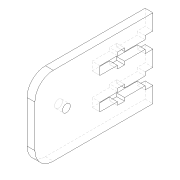
# Autodesk Inventor part: axel mount (3mm shaft)
Saved by Autodesk Inventor 2016 (Build 200138000, 138)
## iProperties
Created: 2014-07-12
Part Number: axel mount (3mm shaft)
Material: Plywood, Finish
Document SubType Name: Modeling
Designer: Sebastian
Density: 0.552 g/cm^3
Appearance: Plywood - New
Description: http://www.wickes.co.uk/Wickes-Non-Structural-Hardwood-Plywood-3-6x607x1829mm/p/110513
Author: Sebastian
Autodesk Inventor part; units mm, degrees
ref_plane "YZ Plane" through (0, 0, 0) normal (1, 0, 0) x (0, 1, 0)
ref_plane "XZ Plane" through (0, 0, 0) normal (0, 1, 0) x (-1, 0, 0)
ref_plane "XY Plane" through (0, 0, 0) normal (0, 0, 1) x (1, 0, 0)
sketch "Sketch1" plane through (0, 0, 0) normal (1, 0, 0) x (0, 1, 0)
  line L0 (0, 0) -> (45, 0)
  line L1 (45, 0) -> (45, -30)
  line L2 (45, -30) -> (0, -30)
  line L3 (0, -30) -> (0, 0)
  dimension "d0" = 45
  dimension "d1" = 30
  constraints: 8 end point, 2 parallel, 1 horizontal, 1 perpendicular
  measures "d0" distance of L1.end L2.end
  measures "d1" distance of L0.end L1.end
extrude "Extrusion1" add sketch "Sketch1" along normal blind 3
sketch "Sketch2" plane through (3, 0, 0) normal (1, 0, 0) x (0, 0, -1)
  line L0 (30, 45) -> (0, 45) projected
  line L1 (6, 45) -> (12, 45)
  line L2 (12, 45) -> (12, 42)
  line L3 (6, 42) -> (6, 45)
  line L4 (0, 45) -> (0, 0) projected
  line L5 (18, 45) -> (24, 45)
  line L6 (24, 45) -> (24, 42)
  line L7 (18, 42) -> (18, 45)
  line L8 (30, 0) -> (30, 45) projected
  line L9 (6, 42) -> (7.4, 42)
  line L10 (7.4, 42) -> (7.4, 34.2)
  line L11 (7.4, 34.2) -> (6.2, 34.2)
  line L12 (6.2, 34.2) -> (6.2, 31.45)
  line L13 (6.2, 31.45) -> (7.4, 31.45)
  line L14 (7.4, 31.45) -> (7.4, 24.8)
  line L15 (7.4, 24.8) -> (10.6, 24.8)
  line L16 (10.6, 24.8) -> (10.6, 31.45)
  line L17 (10.6, 31.45) -> (11.8, 31.45)
  line L18 (11.8, 31.45) -> (11.8, 34.2)
  line L19 (11.8, 34.2) -> (10.6, 34.2)
  line L20 (10.6, 42) -> (12, 42)
  line L21 (10.6, 34.2) -> (10.6, 42)
  line L22 (18, 42) -> (19.4, 42)
  line L23 (19.4, 42) -> (19.4, 34.2)
  line L24 (19.4, 34.2) -> (18.2, 34.2)
  line L25 (18.2, 34.2) -> (18.2, 31.45)
  line L26 (18.2, 31.45) -> (19.4, 31.45)
  line L27 (19.4, 24.8) -> (19.4, 31.45)
  line L28 (19.4, 24.8) -> (22.6, 24.8)
  line L29 (22.6, 24.8) -> (22.6, 31.45)
  line L30 (22.6, 31.45) -> (23.8, 31.45)
  line L31 (23.8, 31.45) -> (23.8, 34.2)
  line L32 (23.8, 34.2) -> (22.6, 34.2)
  line L33 (22.6, 42) -> (24, 42)
  line L34 (22.6, 42) -> (22.6, 34.2)
  dimension "d4" = 6
  dimension "d6" = 6
  dimension "d18" = 6
  dimension "d19" = 3
  dimension "d20" = 6
  dimension "d21" = 6
  dimension "d22" = 1.4
  dimension "d23" = 7.8
  dimension "d24" = 1.2
  dimension "d25" = 2.75
  dimension "d26" = 1.2
  dimension "d27" = 6.65
  dimension "d28" = 3.2
  dimension "d29" = 1.2
  dimension "d30" = 1.4
  dimension "d31" = 1.2
  dimension "d32" = 3.2
  dimension "d33" = 1.2
  dimension "d34" = 20.2
  constraints: 64 end point, 27 point on line, 15 perpendicular, 4 parallel, 3 horizontal
  measures "d4" distance of L2.end L3.start
  measures "d6" distance between parallel lines of L3 L4
  measures "d18" distance of L6.end L7.start
  measures "d19" distance of L5.end L6.end
  measures "d20" distance between parallel lines of L8 L6
  measures "d21" distance between parallel lines of L7 L2
  measures "d22" distance of L3.start L9.end
  measures "d23" distance of L9.end L10.end
  measures "d24" distance of L10.end L11.end
  measures "d25" distance of L11.end L12.end
  measures "d26" distance of L12.end L13.end
  measures "d27" distance of L13.end L14.end
  measures "d28" distance of L14.end L15.end
  measures "d29" distance of L16.end L17.end
  measures "d30" distance of L7.start L22.end
  measures "d31" distance of L23.end L24.end
  measures "d32" distance of L27.start L28.end
  measures "d33" distance of L29.end L30.end
  measures "d34" distance between parallel lines of L15 L0
extrude "Extrusion2" cut sketch "Sketch2" against normal blind 4
fillet "Fillet1" radius 7 2 edges at (1.5, 0, 0) (1.5, 0, -30)
sketch "Sketch3" plane through (3, 0, 0) normal (1, 0, 0) x (0, 0, -1)
  circle A0 centre (15, 12) radius 1.5
  line L0 (0, 45) -> (0, 7) projected
  line L1 (7, 0) -> (23, 0) projected
  point P0 (0, 0)
  dimension "d10" = 3
  dimension "d11" = 15
  dimension "d12" = 12
  constraints: 1 centre point
  measures "d10" diameter of A0
  measures "d11" distance from line of L0 A0.centre
  measures "d12" distance from line of L1 A0.centre
extrude "Extrusion3" cut sketch "Sketch3" against normal blind 4
body "Solid1"
